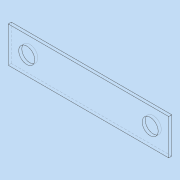
# Autodesk Inventor part: 0 零件
Saved by Autodesk Inventor 2020 (Build 240168000, 168)
## iProperties
Created: 2020-11-03
Part Number: 0 零件
Material: 橡膠
Document SubType Name: Modeling
Designer: p2013
Density: 0.93 g/cm^3
Appearance: 橡膠 - 黑色
Author: p2013
Autodesk Inventor part; units mm, degrees
ref_plane "YZ Plane" through (0, 0, 0) normal (1, 0, 0) x (0, 1, 0)
ref_plane "XZ Plane" through (0, 0, 0) normal (0, 1, 0) x (-1, 0, 0)
ref_plane "XY Plane" through (0, 0, 0) normal (0, 0, 1) x (1, 0, 0)
sketch "草圖1" plane through (0, 0, 0) normal (0, 0, 1) x (1, 0, 0)
  line L0 (0, 0) -> (-50, 0) construction
  line L1 (0, 0) -> (0, 45.4619) construction
  line L2 (-65, -14.5) -> (65, -14.5)
  line L3 (65, -14.5) -> (65, 14.5)
  line L4 (65, 14.5) -> (-65, 14.5)
  line L5 (-65, 14.5) -> (-65, -14.5)
  line L6 (-65, -14.5) -> (65, 14.5) construction
  line L7 (65, -14.5) -> (-65, 14.5) construction
  circle A0 centre (-50, 0) radius 6.5
  circle A1 centre (50, 0) radius 6.5
  dimension "d0" = 29
  dimension "d1" = 130
  dimension "d5" = 13
  dimension "d6" = 100
  constraints: 16 end point, 2 centre point, 2 horizontal, 2 midpoint, 2 parallel, 1 coincident, 1 perpendicular, 1 symmetric about line, 1 vertical, 1 other
  measures "d0" distance between parallel lines of L2 L4
  measures "d1" distance between parallel lines of L3 L5
  measures "d5" diameter of A0
  measures "d6" distance of L0.end A1.centre
extrude "擠出1" add sketch "草圖1" along normal mid plane 2.5
